Autodesk Inventor part; units mm, degrees
(part 2 of 2)
sketch "スケッチ8" plane through (-250, -25, -10) normal (0, -1, 0) x (1, 0, 0)
  line L0 (302, 13.933067) -> (340.076757, 4)
  line L1 (340.076757, 4) -> (302, 4)
  line L2 (302, 4) -> (302, 13.933067)
  line L3 (402, 13.933067) -> (440.076757, 4)
  line L4 (440.076757, 4) -> (402, 4)
  line L5 (402, 4) -> (402, 13.933067)
  line L6 (448, 6.066933) -> (409.923243, 16)
  line L7 (409.923243, 16) -> (448, 16)
  line L8 (448, 16) -> (448, 6.066933)
  line L9 (348, 6.066933) -> (309.923243, 16)
  line L10 (309.923243, 16) -> (348, 16)
  line L11 (348, 16) -> (348, 6.066933)
  line L12 (298, 6.066933) -> (259.923243, 16)
  line L13 (259.923243, 16) -> (298, 16)
  line L14 (298, 16) -> (298, 6.066933)
  line L15 (398, 6.066933) -> (359.923243, 16)
  line L16 (359.923243, 16) -> (398, 16)
  line L17 (398, 16) -> (398, 6.066933)
  line L18 (496, 6.077192) -> (460.624968, 16)
  line L19 (460.624968, 16) -> (496, 16)
  line L20 (496, 16) -> (496, 6.077192)
  line L21 (352, 13.933067) -> (390.076757, 4)
  line L22 (390.076757, 4) -> (352, 4)
  line L23 (352, 4) -> (352, 13.933067)
  line L24 (252, 13.933067) -> (290.076757, 4)
  line L25 (290.076757, 4) -> (252, 4)
  line L26 (252, 4) -> (252, 13.933067)
  line L27 (459.405237, 3.657862) -> (474.609865, 7.922808)
  line L28 (474.609865, 7.922808) -> (489.814493, 3.657862)
  line L29 (489.814493, 3.657862) -> (459.405237, 3.657862)
  line L30 (467.204628, 10) -> (452, 5.735054)
  line L31 (452, 5.735054) -> (452, 14.264946)
  line L32 (452, 14.264946) -> (467.204628, 10)
  line L33 (202, 6.066933) -> (202, 16)
  line L34 (202, 16) -> (240.076757, 16)
  line L35 (240.076757, 16) -> (202, 6.066933)
  line L36 (102, 6.066933) -> (102, 16)
  line L37 (102, 16) -> (140.076757, 16)
  line L38 (140.076757, 16) -> (102, 6.066933)
  line L39 (10.185507, 3.657862) -> (48, 14.264946)
  line L40 (48, 14.264946) -> (48, 3.657862)
  line L41 (48, 3.657862) -> (10.185507, 3.657862)
  line L42 (98, 13.933067) -> (98, 4)
  line L43 (98, 4) -> (90.076757, 4)
  line L44 (90.076757, 4) -> (89.85608, 4.057568)
  line L45 (89.85608, 4.057568) -> (90, 4)
  line L46 (90, 4) -> (59.923243, 4)
  line L47 (59.923243, 4) -> (98, 13.933067)
  line L48 (152, 6.066933) -> (152, 16)
  line L49 (152, 16) -> (190.076757, 16)
  line L50 (190.076757, 16) -> (152, 6.066933)
  line L51 (198, 13.933067) -> (198, 4)
  line L52 (198, 4) -> (159.923243, 4)
  line L53 (159.923243, 4) -> (198, 13.933067)
  line L54 (4, 6.077192) -> (4, 16)
  line L55 (4, 16) -> (39.375032, 16)
  line L56 (39.375032, 16) -> (4, 6.077192)
  line L57 (52, 6.066933) -> (52, 16)
  line L58 (52, 16) -> (59.923243, 16)
  line L59 (59.923243, 16) -> (60.14392, 15.942432)
  line L60 (60.14392, 15.942432) -> (60, 16)
  line L61 (60, 16) -> (90.076757, 16)
  line L62 (90.076757, 16) -> (52, 6.066933)
  line L63 (248, 13.933067) -> (248, 4)
  line L64 (248, 4) -> (209.923243, 4)
  line L65 (209.923243, 4) -> (248, 13.933067)
  line L66 (148, 13.933067) -> (148, 4)
  line L67 (148, 4) -> (109.923243, 4)
  line L68 (109.923243, 4) -> (148, 13.933067)
  line L69 (0, 0) -> (500, 0)
  line L70 (500, 20) -> (500, 0)
  line L71 (500, 20) -> (0, 20)
  line L72 (0, 0) -> (0, 20)
  line L73 (452, 5.735054) -> (452, 3.657862)
  line L74 (452, 4) -> (452, 0)
  line L75 (452, 3.657862) -> (453.656144, 3.657862)
  line L76 (302, 13.933067) -> (340.076757, 4)
  line L77 (340.076757, 4) -> (302, 4)
  line L78 (302, 4) -> (302, 13.933067)
  line L79 (402, 13.933067) -> (440.076757, 4)
  line L80 (440.076757, 4) -> (402, 4)
  line L81 (402, 4) -> (402, 13.933067)
  line L82 (448, 6.066933) -> (409.923243, 16)
  line L83 (409.923243, 16) -> (448, 16)
  line L84 (448, 16) -> (448, 6.066933)
  line L85 (348, 6.066933) -> (309.923243, 16)
  line L86 (309.923243, 16) -> (348, 16)
  line L87 (348, 16) -> (348, 6.066933)
  line L88 (298, 6.066933) -> (259.923243, 16)
  line L89 (259.923243, 16) -> (298, 16)
  line L90 (298, 16) -> (298, 6.066933)
  line L91 (398, 6.066933) -> (359.923243, 16)
  line L92 (359.923243, 16) -> (398, 16)
  line L93 (398, 16) -> (398, 6.066933)
  line L94 (496, 6.077192) -> (460.624968, 16)
  line L95 (460.624968, 16) -> (496, 16)
  line L96 (496, 16) -> (496, 6.077192)
  line L97 (352, 13.933067) -> (390.076757, 4)
  line L98 (390.076757, 4) -> (352, 4)
  line L99 (352, 4) -> (352, 13.933067)
  line L100 (252, 13.933067) -> (290.076757, 4)
  line L101 (290.076757, 4) -> (252, 4)
  line L102 (252, 4) -> (252, 13.933067)
  line L103 (459.405237, 3.657862) -> (474.609865, 7.922808)
  line L104 (474.609865, 7.922808) -> (489.814493, 3.657862)
  line L105 (489.814493, 3.657862) -> (459.405237, 3.657862)
  line L106 (467.204628, 10) -> (452, 5.735054)
  line L107 (452, 5.735054) -> (452, 14.264946)
  line L108 (452, 14.264946) -> (467.204628, 10)
  line L109 (202, 6.066933) -> (202, 16)
  line L110 (202, 16) -> (240.076757, 16)
  line L111 (240.076757, 16) -> (202, 6.066933)
  line L112 (102, 6.066933) -> (102, 16)
  line L113 (102, 16) -> (140.076757, 16)
  line L114 (140.076757, 16) -> (102, 6.066933)
  line L115 (10.185507, 3.657862) -> (48, 14.264946)
  line L116 (48, 14.264946) -> (48, 3.657862)
  line L117 (48, 3.657862) -> (10.185507, 3.657862)
  line L118 (98, 13.933067) -> (98, 4)
  line L119 (98, 4) -> (90.076757, 4)
  line L120 (90.076757, 4) -> (89.85608, 4.057568)
  line L121 (89.85608, 4.057568) -> (90, 4)
  line L122 (90, 4) -> (59.923243, 4)
  line L123 (59.923243, 4) -> (98, 13.933067)
  line L124 (152, 6.066933) -> (152, 16)
  line L125 (152, 16) -> (190.076757, 16)
  line L126 (190.076757, 16) -> (152, 6.066933)
  line L127 (198, 13.933067) -> (198, 4)
  line L128 (198, 4) -> (159.923243, 4)
  line L129 (159.923243, 4) -> (198, 13.933067)
  line L130 (4, 6.077192) -> (4, 16)
  line L131 (4, 16) -> (39.375032, 16)
  line L132 (39.375032, 16) -> (4, 6.077192)
  line L133 (52, 6.066933) -> (52, 16)
  line L134 (52, 16) -> (59.923243, 16)
  line L135 (59.923243, 16) -> (60.14392, 15.942432)
  line L136 (60.14392, 15.942432) -> (60, 16)
  line L137 (60, 16) -> (90.076757, 16)
  line L138 (90.076757, 16) -> (52, 6.066933)
  line L139 (248, 13.933067) -> (248, 4)
  line L140 (248, 4) -> (209.923243, 4)
  line L141 (209.923243, 4) -> (248, 13.933067)
  line L142 (148, 13.933067) -> (148, 4)
  line L143 (148, 4) -> (109.923243, 4)
  line L144 (109.923243, 4) -> (148, 13.933067)
  line L145 (0, 0) -> (500, 0)
  line L146 (500, 20) -> (500, 0)
  line L147 (500, 20) -> (0, 20)
  line L148 (0, 0) -> (0, 20)
  line L149 (302, 13.933067) -> (340.076757, 4)
  line L150 (340.076757, 4) -> (302, 4)
  line L151 (302, 4) -> (302, 13.933067)
  line L152 (402, 13.933067) -> (440.076757, 4)
  line L153 (440.076757, 4) -> (402, 4)
  line L154 (402, 4) -> (402, 13.933067)
  line L155 (448, 6.066933) -> (409.923243, 16)
  line L156 (409.923243, 16) -> (448, 16)
  line L157 (448, 16) -> (448, 6.066933)
  line L158 (348, 6.066933) -> (309.923243, 16)
  line L159 (309.923243, 16) -> (348, 16)
  line L160 (348, 16) -> (348, 6.066933)
  line L161 (298, 6.066933) -> (259.923243, 16)
  line L162 (259.923243, 16) -> (298, 16)
  line L163 (298, 16) -> (298, 6.066933)
  line L164 (398, 6.066933) -> (359.923243, 16)
  line L165 (359.923243, 16) -> (398, 16)
  line L166 (398, 16) -> (398, 6.066933)
  line L167 (496, 6.077192) -> (460.624968, 16)
  line L168 (460.624968, 16) -> (496, 16)
  line L169 (496, 16) -> (496, 6.077192)
  line L170 (352, 13.933067) -> (390.076757, 4)
  line L171 (390.076757, 4) -> (352, 4)
  line L172 (352, 4) -> (352, 13.933067)
  line L173 (252, 13.933067) -> (290.076757, 4)
  line L174 (290.076757, 4) -> (252, 4)
  line L175 (252, 4) -> (252, 13.933067)
  line L176 (459.405237, 3.657862) -> (474.609865, 7.922808)
  line L177 (474.609865, 7.922808) -> (489.814493, 3.657862)
  line L178 (489.814493, 3.657862) -> (459.405237, 3.657862)
  line L179 (467.204628, 10) -> (452, 5.735054)
  line L180 (452, 5.735054) -> (452, 14.264946)
  line L181 (452, 14.264946) -> (467.204628, 10)
  line L182 (202, 6.066933) -> (202, 16)
  line L183 (202, 16) -> (240.076757, 16)
  line L184 (240.076757, 16) -> (202, 6.066933)
  line L185 (102, 6.066933) -> (102, 16)
  line L186 (102, 16) -> (140.076757, 16)
  line L187 (140.076757, 16) -> (102, 6.066933)
  line L188 (10.185507, 3.657862) -> (48, 14.264946)
  line L189 (48, 14.264946) -> (48, 3.657862)
  line L190 (48, 3.657862) -> (10.185507, 3.657862)
  line L191 (98, 13.933067) -> (98, 4)
  line L192 (98, 4) -> (90.076757, 4)
  line L193 (90.076757, 4) -> (89.85608, 4.057568)
  line L194 (89.85608, 4.057568) -> (90, 4)
  line L195 (90, 4) -> (59.923243, 4)
  line L196 (59.923243, 4) -> (98, 13.933067)
  line L197 (152, 6.066933) -> (152, 16)
  line L198 (152, 16) -> (190.076757, 16)
  line L199 (190.076757, 16) -> (152, 6.066933)
  line L200 (198, 13.933067) -> (198, 4)
  line L201 (198, 4) -> (159.923243, 4)
  line L202 (159.923243, 4) -> (198, 13.933067)
  line L203 (4, 6.077192) -> (4, 16)
  line L204 (4, 16) -> (39.375032, 16)
  line L205 (39.375032, 16) -> (4, 6.077192)
  line L206 (52, 6.066933) -> (52, 16)
  line L207 (52, 16) -> (59.923243, 16)
  line L208 (59.923243, 16) -> (60.14392, 15.942432)
  line L209 (60.14392, 15.942432) -> (60, 16)
  line L210 (60, 16) -> (90.076757, 16)
  line L211 (90.076757, 16) -> (52, 6.066933)
  line L212 (248, 13.933067) -> (248, 4)
  line L213 (248, 4) -> (209.923243, 4)
  line L214 (209.923243, 4) -> (248, 13.933067)
  line L215 (148, 13.933067) -> (148, 4)
  line L216 (148, 4) -> (109.923243, 4)
  line L217 (109.923243, 4) -> (148, 13.933067)
  line L218 (0, 0) -> (500, 0)
  line L219 (500, 20) -> (500, 0)
  line L220 (500, 20) -> (0, 20)
  line L221 (0, 0) -> (0, 20)
  line L222 (467.204628, 10) -> (452, 5.735054)
  line L223 (459.405237, 3.657862) -> (474.609865, 7.922808)
  line L224 (467.204628, 10) -> (474.609865, 7.922808)
  line L225 (474.609865, 7.922808) -> (459.405237, 3.657862)
  line L226 (459.405237, 3.657862) -> (474.609865, 7.922808)
  line L227 (452, 5.735054) -> (452, 14.264946)
  line L228 (467.204628, 10) -> (452, 5.735054)
  point P0 (250, 10)
  constraints: 12 end point, 3 collinear, 1 horizontal, 1 parallel, 1 point on line
sketch "スケッチ9" plane through (-250, 25, 10) normal (0, 1, 0) x (1, 0, 0)
  line L0 (190.076757, 4) -> (152, 13.933067)
  line L1 (190.076757, 4) -> (152, 4)
  line L2 (152, 4) -> (152, 13.933067)
  line L3 (89.85608, 15.942432) -> (90.076757, 16)
  line L4 (90.076757, 16) -> (98, 16)
  line L5 (98, 16) -> (98, 6.066933)
  line L6 (59.923243, 16) -> (98, 6.066933)
  line L7 (59.923243, 16) -> (90, 16)
  line L8 (90, 16) -> (89.85608, 15.942432)
  line L9 (39.375032, 4) -> (4, 13.922808)
  line L10 (39.375032, 4) -> (4, 4)
  line L11 (4, 4) -> (4, 13.922808)
  line L12 (140.076757, 4) -> (102, 13.933067)
  line L13 (140.076757, 4) -> (102, 4)
  line L14 (102, 4) -> (102, 13.933067)
  line L15 (240.076757, 4) -> (202, 13.933067)
  line L16 (240.076757, 4) -> (202, 4)
  line L17 (202, 4) -> (202, 13.933067)
  line L18 (159.923243, 16) -> (198, 6.066933)
  line L19 (159.923243, 16) -> (198, 16)
  line L20 (198, 16) -> (198, 6.066933)
  line L21 (60.14392, 4.057568) -> (59.923243, 4)
  line L22 (59.923243, 4) -> (52, 4)
  line L23 (52, 4) -> (52, 13.933067)
  line L24 (90.076757, 4) -> (52, 13.933067)
  line L25 (90.076757, 4) -> (60, 4)
  line L26 (60, 4) -> (60.14392, 4.057568)
  line L27 (109.923243, 16) -> (148, 6.066933)
  line L28 (109.923243, 16) -> (148, 16)
  line L29 (148, 16) -> (148, 6.066933)
  line L30 (209.923243, 16) -> (248, 6.066933)
  line L31 (209.923243, 16) -> (248, 16)
  line L32 (248, 16) -> (248, 6.066933)
  line L33 (474.609865, 12.077192) -> (459.405237, 16.342138)
  line L34 (459.405237, 16.342138) -> (489.814493, 16.342138)
  line L35 (489.814493, 16.342138) -> (474.609865, 12.077192)
  line L36 (452, 5.735054) -> (467.204628, 10)
  line L37 (452, 5.735054) -> (452, 14.264946)
  line L38 (452, 14.264946) -> (467.204628, 10)
  line L39 (10.185507, 16.342138) -> (48, 5.735054)
  line L40 (10.185507, 16.342138) -> (48, 16.342138)
  line L41 (48, 16.342138) -> (48, 5.735054)
  line L42 (0, 0) -> (500, 0)
  line L43 (500, 20) -> (500, 0)
  line L44 (0, 20) -> (500, 20)
  line L45 (0, 0) -> (0, 20)
  line L46 (252, 6.066933) -> (252, 16)
  line L47 (252, 16) -> (290.076757, 16)
  line L48 (252, 6.066933) -> (290.076757, 16)
  line L49 (352, 6.066933) -> (352, 16)
  line L50 (352, 16) -> (390.076757, 16)
  line L51 (352, 6.066933) -> (390.076757, 16)
  line L52 (496, 13.922808) -> (496, 4)
  line L53 (496, 4) -> (460.624968, 4)
  line L54 (496, 13.922808) -> (460.624968, 4)
  line L55 (398, 13.933067) -> (398, 4)
  line L56 (398, 4) -> (359.923243, 4)
  line L57 (398, 13.933067) -> (359.923243, 4)
  line L58 (298, 13.933067) -> (298, 4)
  line L59 (298, 4) -> (259.923243, 4)
  line L60 (298, 13.933067) -> (259.923243, 4)
  line L61 (348, 13.933067) -> (348, 4)
  line L62 (348, 4) -> (309.923243, 4)
  line L63 (348, 13.933067) -> (309.923243, 4)
  line L64 (448, 13.933067) -> (448, 4)
  line L65 (448, 4) -> (409.923243, 4)
  line L66 (448, 13.933067) -> (409.923243, 4)
  line L67 (402, 6.066933) -> (402, 16)
  line L68 (402, 16) -> (440.076757, 16)
  line L69 (402, 6.066933) -> (440.076757, 16)
  line L70 (302, 6.066933) -> (302, 16)
  line L71 (302, 16) -> (340.076757, 16)
  line L72 (302, 6.066933) -> (340.076757, 16)
  line L73 (459.405237, 16.342138) -> (460.624968, 16)
  line L74 (459.405237, 16.342138) -> (451.676498, 16.342138)
  line L75 (451.676498, 16.342138) -> (451.676498, 13.933067)
  line L76 (452, 14.264946) -> (452, 5.735054)
  line L77 (451.676498, 13.933067) -> (452, 14.264946)
  line L78 (452, 14.264946) -> (452, 16.342138)
  line L79 (452, 16) -> (452, 20)
  line L80 (467.204628, 10) -> (452, 14.264946)
  line L81 (452, 14.264946) -> (467.204628, 10)
  line L82 (467.204628, 10) -> (474.609865, 12.077192)
  line L83 (459.405237, 16.342138) -> (474.609865, 12.077192)
  line L84 (459.405237, 16.342138) -> (474.609865, 12.077192)
  point P0 (250, 10)
  constraints: 14 end point, 2 collinear, 2 point on line, 1 horizontal, 1 parallel
sketch "スケッチ9 outline for 押し出し17" plane through (-250, 25, 10) normal (0, 1, 0) x (1, 0, 0)
  line L0 (467.204628, 10) -> (474.609865, 12.077192)
  line L1 (452, 14.264946) -> (467.204628, 10)
  line L2 (452, 16.342138) -> (452, 14.264946)
  line L3 (459.405237, 16.342138) -> (452, 16.342138)
  line L4 (474.609865, 12.077192) -> (459.405237, 16.342138)
extrude "押し出し17" cut sketch "スケッチ9 outline for 押し出し17" against normal through all
sketch "スケッチ10" plane through (-202, -21, -6) normal (-1, 0, 0) x (0, 0, 1)
  line L0 (10.264946, -4) -> (10.264946, 0)
  line L1 (0, 0) -> (10.264946, 0)
  line L2 (0, 42) -> (0, 0)
  line L3 (0, 42) -> (10.264946, 42)
  line L4 (10.264946, 42) -> (10.264946, 46)
  line L5 (-0.342138, 46) -> (10.264946, 46)
  line L6 (-0.342138, 39.235108) -> (-0.342138, 46)
  line L7 (-0.342138, 39.235108) -> (-4, 39.235108)
  line L8 (-4, 0.828427) -> (-4, 39.235108)
  line L9 (-0.342138, 0.828427) -> (-4, 0.828427)
  line L10 (-0.342138, -4) -> (-0.342138, 0.828427)
  line L11 (10.264946, -4) -> (-0.342138, -4)
  point P0 (6, 21)
sketch "スケッチ10 outline for 押し出し18" plane through (-202, -21, -6) normal (-1, 0, 0) x (0, 0, 1)
  line L0 (-0.342138, -4) -> (10.264946, -4)
  line L1 (-0.342138, 0.828427) -> (-0.342138, -4)
  line L2 (-4, 0.828427) -> (-0.342138, 0.828427)
  line L3 (-4, 39.235108) -> (-4, 0.828427)
  line L4 (-0.342138, 39.235108) -> (-4, 39.235108)
  line L5 (-0.342138, 46) -> (-0.342138, 39.235108)
  line L6 (10.264946, 46) -> (-0.342138, 46)
  line L7 (10.264946, 42) -> (10.264946, 46)
  line L8 (0, 42) -> (10.264946, 42)
  line L9 (0, 0) -> (0, 42)
  line L10 (10.264946, 0) -> (0, 0)
  line L11 (10.264946, -4) -> (10.264946, 0)
extrude "押し出し18" add sketch "スケッチ10 outline for 押し出し18" along normal blind 2
sketch "スケッチ11" plane through (-198, -18.291755, -6) normal (1, 0, 0) x (0, 0, -1)
  line L0 (0, 0) -> (0, 36.583509)
  line L1 (0, 0) -> (4, 0)
  line L2 (4, 36.583509) -> (4, 0)
  line L3 (0, 36.583509) -> (4, 36.583509)
  point P0 (-6, 18.291755)
sketch "スケッチ11 outline for 押し出し19" plane through (-198, -18.291755, -6) normal (1, 0, 0) x (0, 0, -1)
  line L0 (0, 0) -> (4, 0)
  line L1 (0, 36.583509) -> (0, 0)
  line L2 (4, 36.583509) -> (0, 36.583509)
  line L3 (4, 0) -> (4, 36.583509)
extrude "押し出し19" cut sketch "スケッチ11 outline for 押し出し19" against normal blind 2
mirror "ミラー3" about plane through (0, 0, 0) normal (0, 0, 1) of "押し出し19", "押し出し18"
sketch "スケッチ12" plane through (-250, -25, 10) normal (0, 0, 1) x (1, 0, 0)
  line L0 (50, 43.291755) -> (52, 43.291755)
  line L1 (52, 43.291755) -> (72.033826, 25)
  line L2 (72.033826, 25) -> (52, 6.708245)
  line L3 (52, 6.708245) -> (50, 6.708245)
  line L4 (50, 6.708245) -> (50, 43.291755)
  line L5 (500, 0) -> (0, 0)
  line L6 (500, 50) -> (500, 0)
  line L7 (0, 50) -> (500, 50)
  line L8 (0, 0) -> (0, 50)
  line L9 (25.520878, 27.307549) -> (6.828427, 46)
  line L10 (6.828427, 46) -> (45.103446, 46)
  line L11 (45.103446, 46) -> (25.520878, 27.307549)
  line L12 (102, 43.291755) -> (122.033826, 25)
  line L13 (122.033826, 25) -> (102, 6.708245)
  line L14 (102, 6.708245) -> (102, 43.291755)
  line L15 (152, 43.291755) -> (172.033826, 25)
  line L16 (172.033826, 25) -> (152, 6.708245)
  line L17 (152, 6.708245) -> (152, 43.291755)
  line L18 (202, 43.291755) -> (222.033826, 25)
  line L19 (222.033826, 25) -> (202, 6.708245)
  line L20 (202, 6.708245) -> (202, 43.291755)
  line L21 (302, 43.291755) -> (322.033826, 25)
  line L22 (322.033826, 25) -> (302, 6.708245)
  line L23 (302, 6.708245) -> (302, 43.291755)
  line L24 (352, 43.291755) -> (372.033826, 25)
  line L25 (372.033826, 25) -> (352, 6.708245)
  line L26 (352, 6.708245) -> (352, 43.291755)
  line L27 (354.966174, 4) -> (375, 22.291755)
  line L28 (375, 22.291755) -> (395.033826, 4)
  line L29 (395.033826, 4) -> (354.966174, 4)
  line L30 (452, 43.235108) -> (471.64993, 24.478357)
  line L31 (471.64993, 24.478357) -> (452, 4.828427)
  line L32 (452, 4.828427) -> (452, 43.235108)
  line L33 (456.828427, 4) -> (474.544134, 21.715707)
  line L34 (474.544134, 21.715707) -> (493.103446, 4)
  line L35 (493.103446, 4) -> (456.828427, 4)
  line L36 (448, 6.708245) -> (427.966174, 25)
  line L37 (427.966174, 25) -> (448, 43.291755)
  line L38 (448, 43.291755) -> (448, 6.708245)
  line L39 (395.033826, 46) -> (375, 27.708245)
  line L40 (375, 27.708245) -> (354.966174, 46)
  line L41 (354.966174, 46) -> (395.033826, 46)
  line L42 (348, 6.708245) -> (327.966174, 25)
  line L43 (327.966174, 25) -> (348, 43.291755)
  line L44 (348, 43.291755) -> (348, 6.708245)
  line L45 (254.966174, 4) -> (275, 22.291755)
  line L46 (275, 22.291755) -> (295.033826, 4)
  line L47 (295.033826, 4) -> (254.966174, 4)
  line L48 (204.966174, 4) -> (225, 22.291755)
  line L49 (225, 22.291755) -> (245.033826, 4)
  line L50 (245.033826, 4) -> (204.966174, 4)
  line L51 (154.966174, 4) -> (175, 22.291755)
  line L52 (175, 22.291755) -> (195.033826, 4)
  line L53 (195.033826, 4) -> (154.966174, 4)
  line L54 (104.966174, 4) -> (125, 22.291755)
  line L55 (125, 22.291755) -> (145.033826, 4)
  line L56 (145.033826, 4) -> (104.966174, 4)
  line L57 (98, 43.291755) -> (98, 6.708245)
  line L58 (98, 6.708245) -> (77.966174, 25)
  line L59 (77.966174, 25) -> (98, 43.291755)
  line L60 (25.455866, 21.715707) -> (43.171573, 4)
  line L61 (43.171573, 4) -> (6.896554, 4)
  line L62 (6.896554, 4) -> (25.455866, 21.715707)
  line L63 (4, 6.764892) -> (4, 43.171573)
  line L64 (4, 43.171573) -> (22.626674, 24.544899)
  line L65 (22.626674, 24.544899) -> (4, 6.764892)
  line L66 (75, 27.708245) -> (54.966174, 46)
  line L67 (54.966174, 46) -> (95.033826, 46)
  line L68 (95.033826, 46) -> (75, 27.708245)
  line L69 (145.033826, 46) -> (125, 27.708245)
  line L70 (125, 27.708245) -> (104.966174, 46)
  line L71 (104.966174, 46) -> (145.033826, 46)
  line L72 (195.033826, 46) -> (175, 27.708245)
  line L73 (175, 27.708245) -> (154.966174, 46)
  line L74 (154.966174, 46) -> (195.033826, 46)
  line L75 (245.033826, 46) -> (225, 27.708245)
  line L76 (225, 27.708245) -> (204.966174, 46)
  line L77 (204.966174, 46) -> (245.033826, 46)
  line L78 (295.033826, 46) -> (275, 27.708245)
  line L79 (275, 27.708245) -> (254.966174, 46)
  line L80 (254.966174, 46) -> (295.033826, 46)
  line L81 (345.033826, 46) -> (325, 27.708245)
  line L82 (325, 27.708245) -> (304.966174, 46)
  line L83 (304.966174, 46) -> (345.033826, 46)
  line L84 (398, 6.708245) -> (377.966174, 25)
  line L85 (377.966174, 25) -> (398, 43.291755)
  line L86 (398, 43.291755) -> (398, 6.708245)
  line L87 (445.033826, 46) -> (425, 27.708245)
  line L88 (425, 27.708245) -> (404.966174, 46)
  line L89 (404.966174, 46) -> (445.033826, 46)
  line L90 (493.171573, 46) -> (474.479122, 27.307549)
  line L91 (474.479122, 27.307549) -> (454.896554, 46)
  line L92 (454.896554, 46) -> (493.171573, 46)
  line L93 (496, 6.764892) -> (477.373326, 24.544899)
  line L94 (477.373326, 24.544899) -> (496, 43.171573)
  line L95 (496, 43.171573) -> (496, 6.764892)
  line L96 (404.966174, 4) -> (425, 22.291755)
  line L97 (425, 22.291755) -> (445.033826, 4)
  line L98 (445.033826, 4) -> (404.966174, 4)
  line L99 (402, 43.291755) -> (422.033826, 25)
  line L100 (422.033826, 25) -> (402, 6.708245)
  line L101 (402, 6.708245) -> (402, 43.291755)
  line L102 (304.966174, 4) -> (325, 22.291755)
  line L103 (325, 22.291755) -> (345.033826, 4)
  line L104 (345.033826, 4) -> (304.966174, 4)
  line L105 (298, 6.708245) -> (277.966174, 25)
  line L106 (277.966174, 25) -> (298, 43.291755)
  line L107 (298, 43.291755) -> (298, 6.708245)
  line L108 (198, 6.708245) -> (177.966174, 25)
  line L109 (177.966174, 25) -> (198, 43.291755)
  line L110 (198, 43.291755) -> (198, 6.708245)
  line L111 (148, 6.708245) -> (127.966174, 25)
  line L112 (127.966174, 25) -> (148, 43.291755)
  line L113 (148, 43.291755) -> (148, 6.708245)
  line L114 (75, 22.291755) -> (95.033826, 4)
  line L115 (95.033826, 4) -> (54.966174, 4)
  line L116 (54.966174, 4) -> (75, 22.291755)
  line L117 (46, 41.326017) -> (46, 6.828427)
  line L118 (46, 6.828427) -> (28.35007, 24.478357)
  line L119 (28.35007, 24.478357) -> (46, 41.326017)
  line L120 (248, 43.291755) -> (248, 6.708245)
  line L121 (248, 6.708245) -> (227.966174, 25)
  line L122 (227.966174, 25) -> (248, 43.291755)
  line L123 (252, 6.708245) -> (252, 43.291755)
  line L124 (252, 43.291755) -> (272.033826, 25)
  line L125 (272.033826, 25) -> (252, 6.708245)
  line L126 (52, 43.291755) -> (72.033826, 25)
  line L127 (52, 43.291755) -> (50, 45.117841)
  line L128 (50, 6.708245) -> (50, 43.291755)
  line L129 (50, 45.117841) -> (50, 43.291755)
  line L130 (250, 25) -> (229.968681, 25)
  line L131 (50, 6.708245) -> (52, 6.708245)
  line L132 (52, 6.708245) -> (50, 4.882159)
  line L133 (50, 4.882159) -> (50, 6.708245)
  constraints: 12 end point, 1 collinear, 1 parallel, 1 point on line, 1 symmetric about line
sketch "スケッチ12 outline for 押し出し20" plane through (-250, -25, 10) normal (0, 0, 1) x (1, 0, 0)
  line L0 (50, 43.291755) -> (52, 43.291755)
  line L1 (50, 45.117841) -> (50, 43.291755)
  line L2 (52, 43.291755) -> (50, 45.117841)
extrude "押し出し20" cut sketch "スケッチ12 outline for 押し出し20" against normal through all
sketch "スケッチ12 outline for 押し出し21" plane through (-250, -25, 10) normal (0, 0, 1) x (1, 0, 0)
  line L0 (50, 6.708245) -> (50, 4.882159)
  line L1 (52, 6.708245) -> (50, 6.708245)
  line L2 (50, 4.882159) -> (52, 6.708245)
extrude "押し出し21" cut sketch "スケッチ12 outline for 押し出し21" against normal through all
sketch "スケッチ13" plane through (-198, 21, 6) normal (1, 0, 0) x (0, 0, -1)
  line L0 (9.933067, 0) -> (9.933067, 4)
  line L1 (0, 4) -> (9.933067, 4)
  line L2 (0, 0) -> (0, 4)
  line L3 (0, 0) -> (9.933067, 0)
  point P0 (6, -21)
sketch "スケッチ14" plane through (-250, 25, 10) normal (0, 1, 0) x (1, 0, 0)
  line L0 (190.076757, 4) -> (152, 13.933067)
  line L1 (190.076757, 4) -> (152, 4)
  line L2 (152, 4) -> (152, 13.933067)
  line L3 (89.85608, 15.942432) -> (90.076757, 16)
  line L4 (90.076757, 16) -> (98, 16)
  line L5 (98, 16) -> (98, 6.066933)
  line L6 (59.923243, 16) -> (98, 6.066933)
  line L7 (59.923243, 16) -> (90, 16)
  line L8 (90, 16) -> (89.85608, 15.942432)
  line L9 (39.375032, 4) -> (4, 13.922808)
  line L10 (39.375032, 4) -> (4, 4)
  line L11 (4, 4) -> (4, 13.922808)
  line L12 (140.076757, 4) -> (102, 13.933067)
  line L13 (140.076757, 4) -> (102, 4)
  line L14 (102, 4) -> (102, 13.933067)
  line L15 (240.076757, 4) -> (202, 13.933067)
  line L16 (240.076757, 4) -> (202, 4)
  line L17 (202, 4) -> (202, 13.933067)
  line L18 (159.923243, 16) -> (198, 6.066933)
  line L19 (159.923243, 16) -> (198, 16)
  line L20 (198, 16) -> (198, 6.066933)
  line L21 (60.14392, 4.057568) -> (59.923243, 4)
  line L22 (59.923243, 4) -> (52, 4)
  line L23 (52, 4) -> (52, 13.933067)
  line L24 (90.076757, 4) -> (52, 13.933067)
  line L25 (90.076757, 4) -> (60, 4)
  line L26 (60, 4) -> (60.14392, 4.057568)
  line L27 (109.923243, 16) -> (148, 6.066933)
  line L28 (109.923243, 16) -> (148, 16)
  line L29 (148, 16) -> (148, 6.066933)
  line L30 (209.923243, 16) -> (248, 6.066933)
  line L31 (209.923243, 16) -> (248, 16)
  line L32 (248, 16) -> (248, 6.066933)
  line L33 (452, 5.735054) -> (489.814493, 16.342138)
  line L34 (452, 5.735054) -> (452, 16.342138)
  line L35 (452, 16.342138) -> (489.814493, 16.342138)
  line L36 (0, 0) -> (500, 0)
  line L37 (500, 20) -> (500, 0)
  line L38 (0, 20) -> (500, 20)
  line L39 (0, 0) -> (0, 20)
  line L40 (252, 6.066933) -> (252, 16)
  line L41 (252, 16) -> (290.076757, 16)
  line L42 (252, 6.066933) -> (290.076757, 16)
  line L43 (352, 6.066933) -> (352, 16)
  line L44 (352, 16) -> (390.076757, 16)
  line L45 (352, 6.066933) -> (390.076757, 16)
  line L46 (496, 13.922808) -> (496, 4)
  line L47 (496, 4) -> (460.624968, 4)
  line L48 (496, 13.922808) -> (460.624968, 4)
  line L49 (398, 13.933067) -> (398, 4)
  line L50 (398, 4) -> (359.923243, 4)
  line L51 (398, 13.933067) -> (359.923243, 4)
  line L52 (298, 13.933067) -> (298, 4)
  line L53 (298, 4) -> (259.923243, 4)
  line L54 (298, 13.933067) -> (259.923243, 4)
  line L55 (348, 13.933067) -> (348, 4)
  line L56 (348, 4) -> (309.923243, 4)
  line L57 (348, 13.933067) -> (309.923243, 4)
  line L58 (448, 13.933067) -> (448, 4)
  line L59 (448, 4) -> (409.923243, 4)
  line L60 (448, 13.933067) -> (409.923243, 4)
  line L61 (402, 6.066933) -> (402, 16)
  line L62 (402, 16) -> (440.076757, 16)
  line L63 (402, 6.066933) -> (440.076757, 16)
  line L64 (302, 6.066933) -> (302, 16)
  line L65 (302, 16) -> (340.076757, 16)
  line L66 (302, 6.066933) -> (340.076757, 16)
  line L67 (46, 6.29606) -> (46, 16.342138)
  line L68 (10.185507, 16.342138) -> (46, 6.29606)
  line L69 (10.185507, 16.342138) -> (46, 16.342138)
  line L70 (52, 4) -> (59.923243, 4)
  line L71 (50, 0) -> (50, 4)
  line L72 (52, 4) -> (50, 4)
  line L73 (50, 4) -> (50, 14.454806)
  line L74 (52, 13.933067) -> (90.076757, 4)
  line L75 (50, 14.454806) -> (52, 13.933067)
  line L76 (52, 13.933067) -> (52, 4)
  point P0 (250, 10)
  constraints: 8 end point, 2 perpendicular, 1 collinear, 1 horizontal
sketch "スケッチ14 outline for 押し出し22" plane through (-250, 25, 10) normal (0, 1, 0) x (1, 0, 0)
  line L0 (52, 13.933067) -> (50, 14.454806)
  line L1 (52, 4) -> (52, 13.933067)
  line L2 (50, 4) -> (52, 4)
  line L3 (50, 14.454806) -> (50, 4)
extrude "押し出し22" cut sketch "スケッチ14 outline for 押し出し22" against normal through all
sketch "スケッチ15" plane through (250, 0, 0) normal (1, 0, 0) x (0, 0, -1)
  line L0 (6, 13.71989) -> (6, -13.71989)
  line L1 (2.080031, 0) -> (6, -13.71989)
  line L2 (6, 13.71989) -> (2.080031, 0)
  line L3 (3.919969, -21) -> (-3.919969, -21)
  line L4 (0, -7.28011) -> (-3.919969, -21)
  line L5 (3.919969, -21) -> (0, -7.28011)
  line L6 (-6, -13.71989) -> (-6, 13.71989)
  line L7 (-2.080031, 0) -> (-6, 13.71989)
  line L8 (-6, -13.71989) -> (-2.080031, 0)
  line L9 (0, 7.28011) -> (3.919969, 21)
  line L10 (-3.919969, 21) -> (0, 7.28011)
  line L11 (-3.919969, 21) -> (3.919969, 21)
  line L12 (-10, -25) -> (10, -25)
  line L13 (10, -25) -> (10, 25)
  line L14 (10, 25) -> (-10, 25)
  line L15 (-10, 25) -> (-10, -25)
  point P0 (0, 0)
sketch "スケッチ15 outline for 押し出し23" plane through (250, 0, 0) normal (1, 0, 0) x (0, 0, -1)
  line L0 (-10, -25) -> (10, -25)
  line L1 (-10, 25) -> (-10, -25)
  line L2 (10, -25) -> (10, 25)
  line L3 (10, 25) -> (-10, 25)
  line L4 (0, -7.28011) -> (3.919969, -21)
  line L5 (-3.919969, -21) -> (0, -7.28011)
  line L6 (3.919969, -21) -> (-3.919969, -21)
  line L7 (-2.080031, 0) -> (-6, -13.71989)
  line L8 (-6, 13.71989) -> (-2.080031, 0)
  line L9 (-6, -13.71989) -> (-6, 13.71989)
  line L10 (2.080031, 0) -> (6, 13.71989)
  line L11 (6, -13.71989) -> (2.080031, 0)
  line L12 (6, 13.71989) -> (6, -13.71989)
  line L13 (-3.919969, 21) -> (3.919969, 21)
  line L14 (0, 7.28011) -> (-3.919969, 21)
  line L15 (3.919969, 21) -> (0, 7.28011)
extrude "押し出し23" cut sketch "スケッチ15 outline for 押し出し23" against normal blind 250
mirror "ミラー4" about plane through (0, 0, 0) normal (1, 0, 0)
